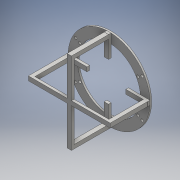
# Autodesk Inventor part: Bottom- Control Surfaces
Saved by Autodesk Inventor 2016 (Build 200138000, 138)
## iProperties
Created: 2016-03-15
Part Number: Bottom- Control Surfaces
Material: Generic
Document SubType Name: Modeling
Designer: s_sud
Density: 1 g/cm^3
Appearance: Default
Author: s_sud
Autodesk Inventor part; units mm, degrees
ref_plane "YZ Plane" through (0, 0, 0) normal (1, 0, 0) x (0, 1, 0)
ref_plane "XZ Plane" through (0, 0, 0) normal (0, 1, 0) x (-1, 0, 0)
ref_plane "XY Plane" through (0, 0, 0) normal (0, 0, 1) x (1, 0, 0)
sketch "Sketch1" plane through (0, 0, 0) normal (0, 1, 0) x (-1, 0, 0)
  circle A0 centre (0, 0) radius 47.5
  circle A1 centre (0, 0) radius 36.5
  dimension "d0" = 95
  dimension "d1" = 73
  constraints: 2 centre point, 2 coincident
  measures "d0" diameter of A0
  measures "d1" diameter of A1
extrude "Extrusion1" add sketch "Sketch1" along normal blind 2
sketch "Sketch4" plane through (0, 0, 0) normal (0, -1, 0) x (1, 0, 0)
  line L0 (-2.5, -22.5) -> (-2.5, -47.5)
  line L1 (-2.5, -47.5) -> (2.5, -47.5)
  line L2 (2.5, -47.5) -> (2.5, -22.5)
  line L3 (2.5, 47.5) -> (-2.5, -47.5) construction
  line L4 (-2.5, 47.5) -> (2.5, -47.5) construction
  line L5 (2.5, -22.5) -> (-2.5, -22.5)
  line L6 (47.5, 2.5) -> (22.5, 2.5)
  line L7 (22.5, -2.5) -> (47.5, -2.5)
  line L8 (22.5, 2.5) -> (22.5, -2.5)
  line L9 (47.5, -2.5) -> (47.5, 2.5)
  line L10 (-2.5, 47.5) -> (-2.5, 22.5)
  line L11 (2.5, 22.5) -> (2.5, 47.5)
  line L12 (-2.5, 22.5) -> (2.5, 22.5)
  line L13 (2.5, 47.5) -> (-2.5, 47.5)
  line L14 (-47.5, -2.5) -> (-22.5, -2.5)
  line L15 (-22.5, 2.5) -> (-47.5, 2.5)
  line L16 (-22.5, -2.5) -> (-22.5, 2.5)
  line L17 (-47.5, 2.5) -> (-47.5, -2.5)
  point P0 (0, 0)
  dimension "d21" = 5
  dimension "d23" = 25
  dimension "d26" = 360
  constraints: 36 end point, 2 midpoint, 1 parallel, 1 perpendicular, 33 other
  measures "d21" distance of L0.end L1.end
  measures "d23" distance between parallel lines of L5 L1
extrude "Extrusion3" add sketch "Sketch4" along normal blind 3
sketch "Sketch5" plane through (0, -3, 0) normal (0, -1, 0) x (1, 0, 0)
  arc A0 (0, -47.5) -> (2.5, -47.4342) centre (0, 0) ccw projected
  line L0 (2.5, -47.4342) -> (-2.5, -47.4342)
  line L1 (-2.5, -47.4342) -> (-2.5, -42.9342)
  line L2 (-2.5, -42.9342) -> (2.5, -42.9342)
  line L3 (2.5, -42.9342) -> (2.5, -47.4342)
  line L4 (47.4342, 2.5) -> (47.4342, -2.5)
  line L5 (47.4342, -2.5) -> (42.9342, -2.5)
  line L6 (42.9342, -2.5) -> (42.9342, 2.5)
  line L7 (42.9342, 2.5) -> (47.4342, 2.5)
  line L8 (-2.5, 47.4342) -> (2.5, 47.4342)
  line L9 (2.5, 47.4342) -> (2.5, 42.9342)
  line L10 (2.5, 42.9342) -> (-2.5, 42.9342)
  line L11 (-2.5, 42.9342) -> (-2.5, 47.4342)
  line L12 (-47.4342, -2.5) -> (-47.4342, 2.5)
  line L13 (-47.4342, 2.5) -> (-42.9342, 2.5)
  line L14 (-42.9342, 2.5) -> (-42.9342, -2.5)
  line L15 (-42.9342, -2.5) -> (-47.4342, -2.5)
  dimension "d30" = 5
  dimension "d31" = 4.5
  dimension "d34" = 360
  constraints: 32 end point, 2 parallel, 1 horizontal, 1 perpendicular, 33 other
  measures "d30" distance of L1.end L2.end
  measures "d31" distance of L0.end L1.end
extrude "Extrusion4" add sketch "Sketch5" along normal blind 40
sketch "Sketch6" plane through (0, -43, 0) normal (0, -1, 0) x (1, 0, 0)
  line L0 (2.5, -36.4143) -> (2.5, -47.4342) projected
  line L1 (-2.5, 36.4143) -> (-2.5, 47.4342) projected
  line L2 (2.5, -47.4342) -> (-2.5, -47.4342)
  line L3 (-2.5, 47.4342) -> (2.5, 47.4342)
  line L4 (36.4143, 2.5) -> (47.4342, 2.5) projected
  line L5 (-47.4342, -2.5) -> (-47.5, -2.5) projected
  line L6 (-47.5, 2.5) -> (-47.5, -2.5)
  line L7 (47.4342, -2.5) -> (47.4342, 2.5)
  line L8 (-47.5, -2.5) -> (-2.5, -2.5)
  line L9 (2.5, -2.5) -> (47.4342, -2.5)
  line L10 (2.5, 47.4342) -> (2.5, 2.5)
  line L11 (2.5, -2.5) -> (2.5, -47.4342)
  line L12 (-2.5, -47.4342) -> (-2.5, -2.5)
  line L13 (-2.5, 2.5) -> (-2.5, 47.4342)
  line L14 (47.4342, 2.5) -> (2.5, 2.5)
  line L15 (-2.5, 2.5) -> (-47.5, 2.5)
  point P0 (0, 0)
  constraints: 24 end point, 10 parallel, 4 perpendicular, 3 horizontal
extrude "Extrusion5" add sketch "Sketch6" along normal blind 3
sketch "Sketch7" plane through (0, 2, 0) normal (0, 1, 0) x (1, 0, 0)
  circle A0 centre (0, -39) radius 1.5
  circle A1 centre (0, -44.5) radius 1.5
  circle A2 centre (38.5381, -22.25) radius 1.5
  circle A3 centre (33.775, -19.5) radius 1.5
  circle A4 centre (38.5381, 22.25) radius 1.5
  circle A5 centre (33.775, 19.5) radius 1.5
  circle A6 centre (0, 44.5) radius 1.5
  circle A7 centre (0, 39) radius 1.5
  circle A8 centre (-38.5381, 22.25) radius 1.5
  circle A9 centre (-33.775, 19.5) radius 1.5
  circle A10 centre (-38.5381, -22.25) radius 1.5
  circle A11 centre (-33.775, -19.5) radius 1.5
  point P0 (0, 0)
  dimension "d41" = 3
  dimension "d42" = 39
  dimension "d43" = 3
  dimension "d44" = 44.5
  dimension "d47" = 360
  constraints: 12 centre point, 25 other
  measures "d41" diameter of A0
  measures "d42" distance of point (0, 0) A0.centre
  measures "d43" diameter of A1
  measures "d44" distance of point (0, 0) A1.centre
extrude "Extrusion6" cut sketch "Sketch7" against normal blind 10 contours A2 | A3 | A4 | A5 | A8 | A9 | A10 | A11
body "Solid1"
